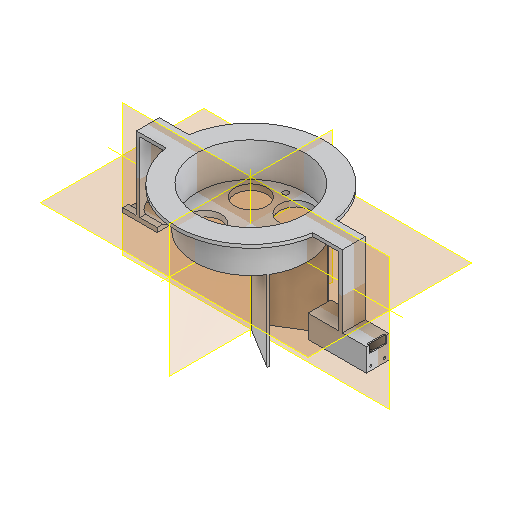
# Autodesk Inventor part: VialHolder
Saved by Autodesk Inventor 2025.1 (Build 291241000, 241)
## iProperties
Created: 2025-05-19
Part Number: VialHolder
Material: Generic
Document SubType Name: Modeling
Designer: Emlyn
Density: 1 g/cm^3
Appearance: Default
Author: Emlyn
Autodesk Inventor part; units mm, degrees
sketch "Sketch1" plane through (0, 0, 0) normal (0, 1, 0) x (-1, 0, 0)
  circle A0 centre (0, 0) radius 49
  dimension "d1" = 98
  constraints: 1 centre point
  measures "d1" diameter of A0
extrude "Extrusion1" add sketch "Sketch1" along normal blind 35
sketch "Sketch4" plane through (0, 35, 0) normal (0, 1, 0) x (1, 0, 0)
  circle A0 centre (0, 0) radius 47
  dimension "d8" = 94
  constraints: 1 centre point, 1 coincident
  measures "d8" diameter of A0
extrude "Extrusion3" cut sketch "Sketch4" against normal blind 30
sketch "Sketch6" plane through (0, 35, 0) normal (0, 1, 0) x (1, 0, 0)
  circle A0 centre (0, 0) radius 49
  circle A1 centre (0, 0) radius 65
  dimension "d13" = 98
  dimension "d14" = 130
  constraints: 2 centre point, 2 coincident
  measures "d13" diameter of A0
  measures "d14" diameter of A1
extrude "Extrusion4" add sketch "Sketch6" against normal blind 3
sketch "Sketch7" plane through (0, 5, 0) normal (0, 1, 0) x (1, 0, 0)
  line L0 (0, 68.6) -> (0, -68.6) projected
  line L1 (68.6, 0) -> (-68.6, 0) projected
  circle A0 centre (29.6304, 0) radius 14
  circle A1 centre (29.6304, 0) radius 15
  circle A2 centre (-20, -20) radius 14
  circle A3 centre (-20, -20) radius 15
  circle A4 centre (12, -27) radius 14
  circle A5 centre (12, -27) radius 15
  circle A6 centre (-20, 20) radius 14
  circle A7 centre (-20, 20) radius 15
  circle A8 centre (12, 27) radius 14
  circle A9 centre (12, 27) radius 15
  circle A10 centre (-7.7127, -37.6577) radius 2.5
  circle A11 centre (40.5942, 15) radius 2.5
  circle A12 centre (-7.7127, 38.4017) radius 2.5
  point P0 (0, 0)
  point P1 (0, -19.7889)
  point P2 (0, -34.2111)
  point P3 (0, 34.2111)
  point P4 (0, 19.7889)
  dimension "d92" = 28
  dimension "d93" = 30
  dimension "d94" = 28
  dimension "d95" = 30
  dimension "d96" = 28
  dimension "d97" = 30
  dimension "d98" = 28
  dimension "d99" = 30
  dimension "d100" = 28
  dimension "d101" = 30
  dimension "d102" = 20
  dimension "d103" = 20
  dimension "d104" = 20
  dimension "d105" = 20
  dimension "d106" = 12
  dimension "d107" = 27
  dimension "d108" = 12
  dimension "d109" = 27
  dimension "d110" = 5
  dimension "d111" = 5
  dimension "d112" = 5
  constraints: 13 centre point, 5 coincident, 1 point on line
  measures "d92" diameter of A0
  measures "d93" diameter of A1
  measures "d94" diameter of A2
  measures "d95" diameter of A3
  measures "d96" diameter of A4
  measures "d97" diameter of A5
  measures "d98" diameter of A6
  measures "d99" diameter of A7
  measures "d100" diameter of A8
  measures "d101" diameter of A9
  measures "d102" distance from line of L1 A6.centre
  measures "d103" distance from line of L1 A2.centre
  measures "d104" distance from line of L0 A6.centre
  measures "d105" distance from line of L0 A3.centre
  measures "d106" distance from line of L0 A8.centre
  measures "d107" distance from line of L1 A8.centre
  measures "d108" distance from line of L0 A4.centre
  measures "d109" distance from line of L1 A4.centre
  measures "d110" diameter of A10
  measures "d111" diameter of A11
  measures "d112" diameter of A12
extrude "Extrusion5" cut sketch "Sketch7" against normal through all contours A8 L0 | L0 A8 | A4 L0 | L0 A4 | A0 L1 | L1 A0 | A2 | A6 | A10 | A11 | A12
sketch "Sketch9" plane through (0, 35, 0) normal (0, 1, 0) x (1, 0, 0)
  circle A0 centre (0, 0) radius 65 projected
  arc A1 (64.2262, -10) -> (64.2262, 10) centre (0, 0) ccw
  line L0 (64.2262, 10) -> (90, 10)
  line L1 (64.2262, -10) -> (90, -10)
  line L2 (90, -10) -> (90, 10)
  line L3 (121, 0) -> (-96, 0) projected
  point P0 (77.1131, 10)
  dimension "d41" = 10
  dimension "d42" = 20
  dimension "d43" = 90
  constraints: 6 end point, 4 point on circle, 2 horizontal, 1 centre point, 1 coincident, 1 midpoint, 1 perpendicular
  measures "d41" distance from line of point (77.113, 10) L3
  measures "d42" distance between parallel lines of L1 L0
  measures "d43" distance from line of A0.centre L2
extrude "Extrusion6" add sketch "Sketch9" against normal blind 3 contours L3 L2 L1 A0 | A0 L0 L2 L3
mirror "Mirror1" about plane through (0, 0, 0) normal (1, 0, 0) of "Extrusion6"
sketch "Sketch10" plane through (0, 32, 0) normal (0, -1, 0) x (1, 0, 0)
  line L0 (-90, 10) -> (-90, -10) projected
  line L1 (-90, 10) -> (-87, 10)
  line L2 (-87, 10) -> (-87, -10)
  line L3 (-87, -10) -> (-90, -10)
  line L4 (-90, -10) -> (-90, 10)
  point P0 (0, 0)
  dimension "d44" = 3
  constraints: 8 end point, 2 parallel, 1 horizontal, 1 perpendicular
  measures "d44" distance between parallel lines of L0 L2
extrude "Extrusion7" add sketch "Sketch10" along normal blind 65
sketch "Sketch12" plane through (-90, 35, -10) normal (-1, 0, 0) x (0, 0, 1)
  circle A0 centre (10, -60) radius 6.5
  line L0 (20, -68) -> (0, -68) projected
  point P0 (10, -35)
  dimension "d49" = 13
  dimension "d50" = 8
  constraints: 1 centre point
  measures "d49" diameter of A0
  measures "d50" distance from line of A0.centre L0
extrude "Extrusion9" cut sketch "Sketch12" against normal blind 3
sketch "Sketch13" plane through (-87, 32, 10) normal (1, 0, 0) x (0, 0, -1)
  circle A0 centre (10, -57) radius 6.5 projected
  arc A1 (5, -61.1533) -> (15, -61.1533) centre (10, -57) ccw
  line L0 (10, -78.6) -> (10, 16.6) projected
  line L1 (5, -61.1533) -> (0, -61.1533)
  line L2 (0, 0) -> (0, -65) projected
  line L3 (20, 0) -> (20, -65) projected
  line L4 (0, -65) -> (20, -65)
  line L5 (20, -65) -> (20, -61.1533)
  line L6 (15, -61.1533) -> (20, -61.1533)
  point P0 (10, -32)
  dimension "d53" = 5
  dimension "d54" = 5
  constraints: 8 end point, 4 point on circle, 3 point on line, 2 horizontal, 1 centre point, 1 coincident
  measures "d53" distance from line of L0 L6.start
  measures "d54" distance from line of L0 L1.start
extrude "Extrusion10" add sketch "Sketch13" along normal blind 15 and the other way blind 15 contours L6 L3 L4 L0 A0 | L0 L4 L2 L1 A0
sketch "Sketch18" plane through (0, 0, 0) normal (0, -1, 0) x (1, 0, 0)
  circle A0 centre (0, 0) radius 49 projected
  circle A1 centre (-20, 20) radius 14 projected
  circle A2 centre (-20, -20) radius 14 projected
  line L0 (10.4184, -6.0653) -> (41.9411, -25.3366)
  line L1 (10.4184, -6.0653) -> (6.9184, -6.0653)
  line L2 (6.9184, -6.0653) -> (40.9681, -26.8814)
  arc A3 (40.8578, 27.0489) -> (39.6703, 28.7622) centre (0, 0) ccw
  arc A4 (40.9681, -26.8814) -> (41.9411, -25.3366) centre (0, 0) ccw
  line L3 (0, 0) -> (49, 0)
  line L4 (10.4184, 6.0653) -> (41.9411, 25.3366)
  line L5 (10.4184, 6.0653) -> (6.9184, 6.0653)
  line L6 (6.9184, 6.0653) -> (40.9681, 26.8814)
  arc A5 (41.9411, 25.3366) -> (40.9681, 26.8814) centre (0, 0) ccw
  dimension "d115" = 3.5
  constraints: 14 end point, 11 point on circle, 4 symmetric about line, 3 centre point, 3 coincident, 1 horizontal, 1 parallel
  measures "d115" distance of L0.start L1.end
extrude "Extrusion15" add sketch "Sketch18" along normal blind 70 contours L4 L5 L6 A0 | A0 L2 L1 L0
sketch "Sketch19" plane through (0, 32, 0) normal (0, -1, 0) x (1, 0, 0)
  line L0 (90, -10) -> (64.2262, -10) projected
  line L1 (90, 10) -> (87, 10)
  line L2 (87, 10) -> (87, -10)
  line L3 (87, -10) -> (90, -10)
  line L4 (90, -10) -> (90, 10)
  point P0 (0, 0)
  dimension "d118" = 3
  constraints: 8 end point, 2 parallel, 1 horizontal, 1 perpendicular, 1 point on line
  measures "d118" distance of L3.end L2.end
extrude "Extrusion16" add sketch "Sketch19" along normal blind 80
sketch "Sketch20" plane through (90, 35, 10) normal (1, 0, 0) x (0, 0, -1)
  line L0 (0, -3) -> (0, -64.1533) projected
  line L1 (20, 0) -> (20, -83) projected
  line L2 (0, -63) -> (20, -63)
  line L3 (20, -63) -> (20, -83)
  line L4 (20, -83) -> (0, -83)
  line L5 (0, -83) -> (0, -63)
  line L6 (1, -64) -> (19, -64)
  line L7 (19, -64) -> (19, -82)
  line L8 (19, -82) -> (1, -82)
  line L9 (1, -82) -> (1, -64)
  point P0 (10, -35)
  dimension "d121" = 20
  dimension "d122" = 18
  dimension "d123" = 18
  dimension "d124" = 19
  dimension "d125" = 1
  constraints: 16 end point, 4 parallel, 2 horizontal, 2 perpendicular, 1 point on line
  measures "d121" distance between parallel lines of L4 L2
  measures "d122" distance of L6.start L6.end
  measures "d123" distance of L6.end L7.end
  measures "d124" distance between parallel lines of L4 L6
  measures "d125" distance between parallel lines of L5 L9
extrude "Extrusion17" cut sketch "Sketch20" against normal blind 3 contours L6 L7 L8 L9
sketch "Sketch21" plane through (90, 35, 10) normal (1, 0, 0) x (0, 0, -1)
  line L0 (19, -64) -> (1, -64) projected
  line L1 (19, -82) -> (19, -64) projected
  line L2 (1, -64) -> (19, -64)
  line L3 (19, -64) -> (19, -82)
  line L4 (19, -82) -> (1, -82)
  line L5 (1, -82) -> (1, -64)
  line L6 (0, -3) -> (0, -83) projected
  line L7 (0, -83) -> (20, -83) projected
  line L8 (0, -63) -> (20, -63)
  line L9 (20, -63) -> (20, -83)
  line L10 (20, -83) -> (0, -83)
  line L11 (0, -83) -> (0, -63)
  point P0 (10, -35)
  dimension "d128" = 20
  constraints: 16 end point, 4 parallel, 2 horizontal, 2 perpendicular, 1 point on line
  measures "d128" distance of L8.end L7.end
extrude "Extrusion18" add sketch "Sketch21" along normal blind 20 and the other way blind 30
sketch "Sketch22" plane through (110, 35, 10) normal (1, 0, 0) x (0, 0, -1)
  line L0 (0, -63) -> (20, -63) projected
  line L1 (20, -63) -> (20, -83) projected
  line L2 (0, -63) -> (20, -63)
  line L3 (20, -63) -> (20, -83)
  line L4 (20, -83) -> (0, -83)
  line L5 (0, -83) -> (0, -63)
  point P0 (10, -35)
  constraints: 8 end point, 2 parallel, 1 horizontal, 1 perpendicular
extrude "Extrusion19" add sketch "Sketch22" along normal blind 1
sketch "Sketch23" plane through (111, 35, 10) normal (1, 0, 0) x (0, 0, -1)
  line L0 (2.5, -65.5) -> (17.5, -65.5)
  line L1 (17.5, -65.5) -> (17.5, -69.5)
  line L2 (17.5, -69.5) -> (2.5, -69.5)
  line L3 (2.5, -69.5) -> (2.5, -65.5)
  line L4 (10, -126) -> (10, 21) projected
  line L5 (0, -83) -> (20, -83) projected
  circle A0 centre (16, -79.5) radius 1
  line L6 (20, -83) -> (20, -63) projected
  circle A1 centre (4, -79.5) radius 1
  line L7 (0, -63) -> (0, -83) projected
  point P0 (10, -35)
  point P1 (17.5, -67.5)
  dimension "d135" = 15
  dimension "d136" = 7.5
  dimension "d137" = 4
  dimension "d138" = 17.5
  dimension "d139" = 10
  dimension "d140" = 2
  dimension "d141" = 4
  dimension "d142" = 2
  dimension "d143" = 10
  dimension "d144" = 4
  constraints: 8 end point, 2 centre point, 2 parallel, 1 horizontal, 1 midpoint, 1 perpendicular
  measures "d135" distance of L1.end L2.end
  measures "d136" distance from line of L4 point (17.5, -67.5)
  measures "d137" distance of L0.end L1.end
  measures "d138" distance between parallel lines of L5 L0
  measures "d139" distance from line of L2 A0.centre
  measures "d140" diameter of A0
  measures "d141" distance from line of L6 A0.centre
  measures "d142" diameter of A1
  measures "d143" distance from line of A1.centre L2
  measures "d144" distance from line of L7 A1.centre
extrude "Extrusion20" cut sketch "Sketch23" against normal blind 1
sketch "Sketch24" plane through (90, -28, 10) normal (0, 1, 0) x (1, 0, 0)
  line L0 (21, 20) -> (21, 0) projected
  line L1 (19, 17.5) -> (21, 17.5)
  line L2 (21, 17.5) -> (21, 2.5)
  line L3 (21, 2.5) -> (19, 2.5)
  line L4 (19, 2.5) -> (19, 17.5)
  line L5 (0, 0) -> (21, 0) projected
  point P0 (-90, 10)
  dimension "d147" = 15
  dimension "d148" = 2.5
  dimension "d149" = 2
  constraints: 8 end point, 2 parallel, 1 horizontal, 1 perpendicular, 1 point on line
  measures "d147" distance of L3.end L1.start
  measures "d148" distance from line of L5 L3.end
  measures "d149" distance between parallel lines of L0 L4
extrude "Extrusion21" cut sketch "Sketch24" against normal blind 4
body "Solid1"
